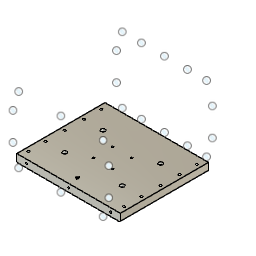
CAD_File 6 (Autodesk Fusion 360 design; units mm, degrees)
Autodesk Fusion 360 part; units mm, degrees
sketch "Sketch1" plane through (0, 0, -172.35) normal (0, 0, -1) x (1, 0, 0)
  line L0 (135, -115) -> (135, 115)
  line L1 (135, 115) -> (115, 115)
  line L2 (115, 115) -> (115, -115)
  line L3 (115, -115) -> (135, -115)
  line L4 (-135, -115) -> (135, -115)
  line L5 (-135, 115) -> (-135, -115)
  line L6 (135, -115) -> (135, 115)
  line L7 (135, 115) -> (-135, 115)
extrude "Extrude1" add sketch "Sketch1" along normal blind 20
chamfer "Chamfer1" distance 2 angle 45 2 edges at (-135, 0, -192.35) (135, 0, -192.35)
sketch "Sketch2" plane through (0, 0, -192.35) normal (0, 0, -1) x (1, 0, 0)
  line L0 (133, -115) -> (133, 115)
  line L1 (133, 115) -> (-133, 115)
  line L2 (-133, 115) -> (-133, -115)
  line L3 (-133, -115) -> (133, -115)
  circle A0 centre (-125, 95) radius 3
  circle A1 centre (-125, 95) radius 5.5
  circle A2 centre (-125, 50) radius 3
  circle A3 centre (-125, 0) radius 3
  circle A4 centre (-125, 0) radius 5.5
  circle A5 centre (-125, -50) radius 3
  circle A6 centre (-125, -95) radius 3
  circle A7 centre (-125, -95) radius 5.5
  circle A8 centre (125, -95) radius 5.5
  circle A9 centre (125, -95) radius 3
  circle A10 centre (125, -50) radius 3
  circle A11 centre (125, 0) radius 3
  circle A12 centre (125, 0) radius 5.5
  circle A13 centre (125, 50) radius 3
  circle A14 centre (125, 95) radius 3
  circle A15 centre (125, 95) radius 5.5
extrude "Extrude2" cut sketch "Sketch2" against normal blind 40 contours A0 | A3 | A6 | A9 | A11 | A14
extrude "Extrude3" cut sketch "Sketch2" against normal blind 35 contours A2 | A5 | A10 | A13
extrude "Extrude4" cut sketch "Sketch2" against normal blind 6.5 contours A1 | A4 | A7 | A8 | A12 | A15
sketch "sketch 2431" plane through (0, 135, 0) normal (0, 1, 0) x (-1, 0, 0)
  circle A0 centre (-110, -182.35) radius 3
  circle A1 centre (110, -182.35) radius 3
  circle A2 centre (125, -60) radius 3
  circle A3 centre (0, -10) radius 3
  circle A4 centre (-125, -60) radius 3
  circle A5 centre (-110, -10) radius 3
  circle A6 centre (110, -10) radius 3
  circle A7 centre (125, -132.35) radius 3
  circle A8 centre (0, -182.35) radius 3
  circle A9 centre (-125, -132.35) radius 3
extrude "Extrude5" cut sketch "sketch 2431" against normal blind 40
sketch "sketch 2480" plane through (0, 135, 0) normal (0, 1, 0) x (-1, 0, 0)
  circle A0 centre (-60, -10) radius 3
  circle A1 centre (-60, -182.35) radius 3
  circle A2 centre (60, -182.35) radius 3
  circle A3 centre (60, -10) radius 3
extrude "Extrude6" cut sketch "sketch 2480" against normal blind 35
sketch "sketch 2504" plane through (0, -135, 0) normal (0, -1, 0) x (1, 0, 0)
  circle A0 centre (-110, -182.35) radius 3
  circle A1 centre (110, -182.35) radius 3
  circle A2 centre (125, -60) radius 3
  circle A3 centre (0, -10) radius 3
  circle A4 centre (-125, -60) radius 3
  circle A5 centre (-110, -10) radius 3
  circle A6 centre (110, -10) radius 3
  circle A7 centre (125, -132.35) radius 3
  circle A8 centre (0, -182.35) radius 3
  circle A9 centre (-125, -132.35) radius 3
extrude "Extrude7" cut sketch "sketch 2504" against normal blind 40
thread "Thread1" "ISO Metric profile 6.0 M6x1 6H" major diameter 6.147 minor diameter 5.035 pitch 1 angle 60 resizes the face on face at (-107.0595, -101.6667, -181.7556) on face at (2.8191, -101.6667, -181.3239) on face at (112.9405, -101.6667, -181.7556) on face at (107.0595, 101.6667, -181.7556) on face at (-2.8191, 101.6667, -181.3239) on face at (-112.9405, 101.6667, -181.7556)
sketch "Sketch3" plane through (0, 0, -172.35) normal (0, 0, 1) x (-1, 0, 0)
  circle A0 centre (-125, 50) radius 3
  circle A1 centre (125, -50) radius 3
  circle A2 centre (-125, -50) radius 3
  circle A3 centre (125, 50) radius 3
  circle A4 centre (-125, 95) radius 3
  circle A5 centre (125, -95) radius 3
  circle A6 centre (-125, 0) radius 3
  circle A7 centre (125, 95) radius 3
  circle A8 centre (125, 0) radius 3
  circle A9 centre (-125, -95) radius 3
  line L0 (135, 115) -> (-135, 115)
  line L1 (-135, 115) -> (-135, -115)
  line L2 (-135, -115) -> (135, -115)
  line L3 (135, -115) -> (135, 115)
  line L4 (150, 0) -> (-150, 0) construction
  line L5 (0, -125) -> (0, 125) construction
  circle A10 centre (75, -50) radius 3.1
  circle A11 centre (75, -50) radius 5.5
  circle A12 centre (-75, -50) radius 3.1
  circle A13 centre (-75, -50) radius 5.5
  circle A14 centre (75, 50) radius 5.5
  circle A15 centre (75, 50) radius 3.1
  circle A16 centre (-75, 50) radius 3.1
  circle A17 centre (-75, 50) radius 5.5
  circle A18 centre (25, -25) radius 3
  circle A19 centre (-25, -25) radius 3
  circle A20 centre (25, 25) radius 3
  circle A21 centre (-25, 25) radius 3
  dimension "d628" = 6.2
  dimension "d629" = 50
  dimension "d630" = 75
  dimension "d631" = 11
  dimension "d636" = 6
  dimension "d637" = 25
  dimension "d638" = 25
  constraint horizontal L4
  constraint perpendicular L2 L5
  constraint concentric A10 A11
  constraint symmetric L5 A10 A12
  constraint symmetric L5 A11 A13
  constraint symmetric L4 A10 A15
  constraint symmetric L4 A11 A14
  constraint symmetric L4 A12 A16
  constraint symmetric L4 A13 A17
  constraint symmetric L5 A18 A19
  constraint symmetric L4 A18 A20
  constraint symmetric L4 A19 A21
  measures "d628" diameter of A10
  measures "d629" distance of L4 A10.centre
  measures "d630" distance of L5 A10.centre
  measures "d631" diameter of A11
  measures "d636" diameter of A18
  measures "d637" distance of L5 A18.centre
  measures "d638" distance of L4 A18.centre
extrude "Extrude10" cut sketch "Sketch3" against normal up to surface (20 mm away) contours A18 | A19 | A20 | A21
extrude "Extrude8" cut sketch "Sketch3" against normal up to surface (20 mm away) contours A10 | A12 | A15 | A16
extrude "Extrude9" cut sketch "Sketch3" against normal blind 6.5 contours A11 | A13 | A14 | A17
thread "Thread2" "ISO Metric profile 6.0 M6x1 6H" major diameter 6.147 minor diameter 5.035 pitch 1 angle 60 resizes the face on face at (-27.9963, 25.1495, -185.6833) on face at (-27.9963, -24.8505, -185.6833) on face at (22.0037, 25.1495, -185.6833) on face at (22.0037, -24.8505, -185.6833)
sketch "Sketch4" plane through (0, 0, -172.35) normal (0, 0, 1) x (-1, 0, 0)
  circle A0 centre (-75, -50) radius 5.5
  circle A1 centre (-75, 50) radius 5.5
  circle A2 centre (75, -50) radius 5.5
  circle A3 centre (75, 50) radius 5.5
  circle A4 centre (-25, -25) radius 2.5175
  circle A5 centre (-25, 25) radius 2.5175
  circle A6 centre (25, -25) radius 2.5175
  circle A7 centre (25, 25) radius 2.5175
  circle A8 centre (-125, 50) radius 3
  circle A9 centre (125, -50) radius 3
  circle A10 centre (-125, -50) radius 3
  circle A11 centre (125, 50) radius 3
  circle A12 centre (-125, 95) radius 3
  circle A13 centre (125, -95) radius 3
  circle A14 centre (-125, 0) radius 3
  circle A15 centre (125, 95) radius 3
  circle A16 centre (125, 0) radius 3
  circle A17 centre (-125, -95) radius 3
  line L0 (135, 115) -> (-135, 115)
  line L1 (-135, 115) -> (-135, -115)
  line L2 (-135, -115) -> (135, -115)
  line L3 (135, -115) -> (135, 115)
  line L4 (0.6617, 95) -> (0.6617, 92.6057)
  line L5 (0.6617, 92.6057) -> (5, 92.6057)
  line L6 (5, 92.6057) -> (5, 91.4802)
  line L7 (5, 91.4802) -> (0.4366, 85)
  line L8 (0.4366, 85) -> (-0.5662, 85)
  line L9 (-0.5662, 85) -> (-0.5662, 91.4802)
  line L10 (-0.5662, 91.4802) -> (-1.9168, 91.4802)
  line L11 (-1.9168, 91.4802) -> (-1.9168, 92.6057)
  line L12 (-1.9168, 92.6057) -> (-0.5662, 92.6057)
  line L13 (-0.5662, 92.6057) -> (-0.5662, 95)
  line L14 (-0.5662, 95) -> (0.6617, 95)
  line L15 (0.6617, 91.4802) -> (0.6617, 86.9714)
  line L16 (0.6617, 86.9714) -> (3.7926, 91.4802)
  line L17 (3.7926, 91.4802) -> (0.6617, 91.4802)
extrude "Extrude11" cut sketch "Sketch4" against normal blind 0.2 contours L4 L5 L6 L7 L8 L9 L10 L11 L12 L13 L14
